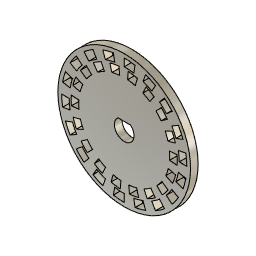
_Encoder Wheel.eb9523d5-e484-4a40-b553-a28b88c10ead (Autodesk Fusion 360 design; units mm, degrees)
Autodesk Fusion 360 part; units mm, degrees
sketch "Sketch1" plane through (0, 0, 0) normal (0, 1, 0) x (1, 0, 0)
  circle A0 centre (0, 0) radius 12
  line L0 (0, 0) -> (0, -7.9531) construction
  line L1 (0.88, -11.9677) -> (1.0543, -13.9601)
  circle A1 centre (0, 0) radius 13.9998
  circle A2 centre (0, 0) radius 14.4998
  line L2 (0, -14.4998) -> (0, -16.4998)
  circle A3 centre (0, 0) radius 16.4998
  circle A4 centre (0, 0) radius 17.4998
  line L3 (2.5179, -14.2796) -> (2.8652, -16.2492)
  line L4 (2.9448, -11.6331) -> (3.4624, -13.5649)
  line L5 (4.9592, -13.6254) -> (5.6433, -15.5048)
  line L6 (4.9201, -10.945) -> (5.7654, -12.7576)
  line L7 (7.2499, -12.5572) -> (8.2499, -14.2893)
  line L8 (6.7459, -9.9243) -> (7.8931, -11.5626)
  line L9 (9.3203, -11.1075) -> (10.6059, -12.6396)
  line L10 (8.3668, -8.6021) -> (9.781, -10.0163)
  line L11 (11.1075, -9.3203) -> (12.6396, -10.6059)
  line L12 (9.7334, -7.0186) -> (11.3717, -8.1657)
  line L13 (12.5572, -7.2499) -> (14.2893, -8.2499)
  line L14 (10.8043, -5.2217) -> (12.6169, -6.067)
  line L15 (13.6254, -4.9592) -> (15.5048, -5.6433)
  line L16 (11.5469, -3.2663) -> (13.4788, -3.7839)
  line L17 (14.2796, -2.5179) -> (16.2492, -2.8652)
  line L18 (11.9387, -1.2115) -> (13.9311, -1.3858)
  line L19 (14.4998, 0) -> (16.4998, 0)
  line L20 (11.9677, 0.88) -> (13.9601, 1.0543)
  line L21 (14.2796, 2.5179) -> (16.2492, 2.8652)
  line L22 (11.6331, 2.9448) -> (13.5649, 3.4624)
  line L23 (13.6254, 4.9592) -> (15.5048, 5.6433)
  line L24 (10.945, 4.9201) -> (12.7576, 5.7654)
  line L25 (12.5572, 7.2499) -> (14.2893, 8.2499)
  line L26 (9.9243, 6.7459) -> (11.5626, 7.8931)
  line L27 (11.1075, 9.3203) -> (12.6396, 10.6059)
  line L28 (8.6021, 8.3668) -> (10.0163, 9.781)
  line L29 (9.3203, 11.1075) -> (10.6059, 12.6396)
  line L30 (7.0186, 9.7334) -> (8.1657, 11.3717)
  line L31 (7.2499, 12.5572) -> (8.2499, 14.2893)
  line L32 (5.2217, 10.8043) -> (6.067, 12.6169)
  line L33 (4.9592, 13.6254) -> (5.6433, 15.5048)
  line L34 (3.2663, 11.5469) -> (3.7839, 13.4788)
  line L35 (2.5179, 14.2796) -> (2.8652, 16.2492)
  line L36 (1.2115, 11.9387) -> (1.3858, 13.9311)
  line L37 (0, 14.4998) -> (0, 16.4998)
  line L38 (-0.88, 11.9677) -> (-1.0543, 13.9601)
  line L39 (-2.5179, 14.2796) -> (-2.8652, 16.2492)
  line L40 (-2.9448, 11.6331) -> (-3.4624, 13.5649)
  line L41 (-4.9592, 13.6254) -> (-5.6433, 15.5048)
  line L42 (-4.9201, 10.945) -> (-5.7654, 12.7576)
  line L43 (-7.2499, 12.5572) -> (-8.2499, 14.2893)
  line L44 (-6.7459, 9.9243) -> (-7.8931, 11.5626)
  line L45 (-9.3203, 11.1075) -> (-10.6059, 12.6396)
  line L46 (-8.3668, 8.6021) -> (-9.781, 10.0163)
  line L47 (-11.1075, 9.3203) -> (-12.6396, 10.6059)
  line L48 (-9.7334, 7.0186) -> (-11.3717, 8.1657)
  line L49 (-12.5572, 7.2499) -> (-14.2893, 8.2499)
  line L50 (-10.8043, 5.2217) -> (-12.6169, 6.067)
  line L51 (-13.6254, 4.9592) -> (-15.5048, 5.6433)
  line L52 (-11.5469, 3.2663) -> (-13.4788, 3.7839)
  line L53 (-14.2796, 2.5179) -> (-16.2492, 2.8652)
  line L54 (-11.9387, 1.2115) -> (-13.9311, 1.3858)
  line L55 (-14.4998, 0) -> (-16.4998, 0)
  line L56 (-11.9677, -0.88) -> (-13.9601, -1.0543)
  line L57 (-14.2796, -2.5179) -> (-16.2492, -2.8652)
  line L58 (-11.6331, -2.9448) -> (-13.5649, -3.4624)
  line L59 (-13.6254, -4.9592) -> (-15.5048, -5.6433)
  line L60 (-10.945, -4.9201) -> (-12.7576, -5.7654)
  line L61 (-12.5572, -7.2499) -> (-14.2893, -8.2499)
  line L62 (-9.9243, -6.7459) -> (-11.5626, -7.8931)
  line L63 (-11.1075, -9.3203) -> (-12.6396, -10.6059)
  line L64 (-8.6021, -8.3668) -> (-10.0163, -9.781)
  line L65 (-9.3203, -11.1075) -> (-10.6059, -12.6396)
  line L66 (-7.0186, -9.7334) -> (-8.1657, -11.3717)
  line L67 (-7.2499, -12.5572) -> (-8.2499, -14.2893)
  line L68 (-5.2217, -10.8043) -> (-6.067, -12.6169)
  line L69 (-4.9592, -13.6254) -> (-5.6433, -15.5048)
  line L70 (-3.2663, -11.5469) -> (-3.7839, -13.4788)
  line L71 (-2.5179, -14.2796) -> (-2.8652, -16.2492)
  line L72 (-1.2115, -11.9387) -> (-1.3858, -13.9311)
  circle A5 centre (0, 0) radius 2.6
  circle A6 centre (0, 0) radius 2
  line L73 (-1.6613, -2) -> (1.6613, -2)
  dimension "d1" = 24
  dimension "d6" = 27.9997
  dimension "d16" = 360
  dimension "d20" = 5.2
  dimension "d21" = 0.5
  dimension "d22" = 1
  dimension "d23" = 5
  dimension "d24" = 0.88
  dimension "d25" = 2
  dimension "d26" = 2
  dimension "d27" = 34.9997
  dimension "d28" = 4
  constraint coincident A0.centre L0.start
  constraint vertical L0
  constraint coincident A0 L1.start
  constraint concentric A0 A1
  constraint coincident L1.end A1
  constraint concentric A1 A2
  constraint coincident A2 L2.start
  constraint vertical L2
  constraint concentric A2 A3
  constraint concentric A1 A4
  constraint coincident L2.end A3
  constraint collinear L0 L2
  constraint concentric A4 A5
  constraint concentric A2 A6
  constraint coincident A5 L73.start
  constraint tangent A6 L73
  constraint horizontal L73
  constraint coincident A5 L73.end
  measures "d1" diameter of A0
  measures "d6" diameter of A1
  measures "d20" diameter of A5
  measures "d21" distance of A1 A2
  measures "d22" distance of A3 A4
  measures "d23" angle of L0 L1
  measures "d24" distance of L0 L1.start
  measures "d25" distance of L1.start L1.end
  measures "d26" distance of L2.start L2.end
  measures "d27" diameter of A4
  measures "d28" diameter of A6
extrude "Extrude1" add sketch "Sketch1" along normal blind 2 contours A0 | A0 A1 L20 L22 | A0 A1 L16 L18 | A0 A1 L24 L26 | A0 A1 L12 L14 | A0 A1 L28 L30 | A0 A1 L8 L10 | A0 A1 L32 L34 | A0 A1 L4 L6 | A0 A1 L36 L38 | A0 L1 A1 L72 | A0 A1 L40 L42 | A0 A1 L68 L70 | A0 A1 L44 L46 | A0 A1 L64 L66 | A0 A1 L48 L50 | A0 A1 L60 L62 | A0 A1 L52 L54 | A0 A1 L56 L58 | A2 | A2 A3 L19 L21 | A2 A3 L15 L17 | A2 A3 L23 L25 | A2 A3 L11 L13 | A2 A3 L27 L29 | A2 A3 L7 L9 | A2 A3 L31 L33 | A2 A3 L3 L5 | A2 A3 L35 L37 | A2 L2 A3 L71 | A2 A3 L39 L41 | A2 A3 L67 L69 | A2 A3 L43 L45 | A2 A3 L63 L65 | A2 A3 L47 L49 | A2 A3 L59 L61 | A2 A3 L51 L53 | A2 A3 L55 L57 | A4 | A5 L73 picked at (0.1198, -2.3917)
convert_to_sheet_metal "ConvertToSheetMetal1"
